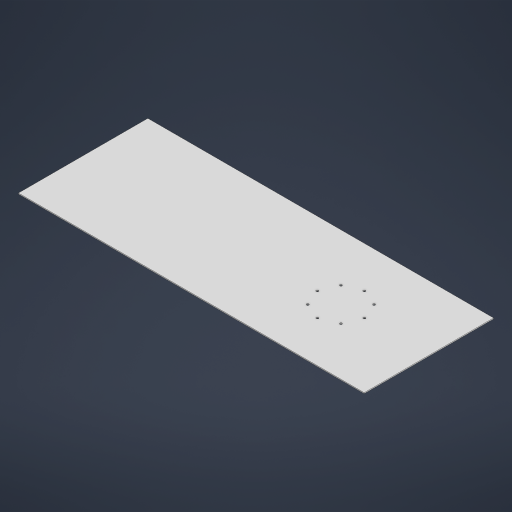
# Autodesk Inventor part: ChassisTop V3
Saved by Autodesk Inventor 2024 (Build 280153000, 153)
## iProperties
Created: 2023-11-20
Part Number: ChassisTop V3
Material: Generic
Document SubType Name: Modeling
Designer: avsar
Density: 1 g/cm^3
Appearance: Default
Author: avsar
Autodesk Inventor part; units mm, degrees
ref_plane "YZ Plane" through (0, 0, 0) normal (1, 0, 0) x (0, 1, 0)
ref_plane "XZ Plane" through (0, 0, 0) normal (0, 1, 0) x (-1, 0, 0)
ref_plane "XY Plane" through (0, 0, 0) normal (0, 0, 1) x (1, 0, 0)
sketch "Sketch1" plane through (0, 0, 0) normal (0, 1, 0) x (-1, 0, 0)
  line L0 (-305.435, 114.3) -> (305.435, 114.3)
  line L1 (305.435, 114.3) -> (305.435, -114.3)
  line L2 (305.435, -114.3) -> (-305.435, -114.3)
  line L3 (-305.435, -114.3) -> (-305.435, 114.3)
  line L4 (-305.435, 114.3) -> (305.435, -114.3) construction
  line L5 (305.435, 114.3) -> (-305.435, -114.3) construction
  point P0 (0, 0)
  dimension "d0" = 610.87
  dimension "d1" = 228.6
  constraints: 12 end point, 2 midpoint, 2 parallel, 1 horizontal, 1 perpendicular
  measures "d0" distance of L1.end L2.end
  measures "d1" distance of L0.end L1.end
extrude "Extrusion1" add sketch "Sketch1" along normal mid plane 1.5875
sketch "Sketch2" plane through (0, 0.7937, 0) normal (0, 1, 0) x (1, 0, 0)
  circle A0 centre (150, 0) radius 41.5 construction
  circle A1 centre (150, 41.5) radius 2
  circle A2 centre (120.6551, 29.3449) radius 2
  circle A3 centre (108.5, 0) radius 2
  circle A4 centre (120.6551, -29.3449) radius 2
  circle A5 centre (150, -41.5) radius 2
  circle A6 centre (179.3449, -29.3449) radius 2
  circle A7 centre (191.5, 0) radius 2
  circle A8 centre (179.3449, 29.3449) radius 2
  point P0 (0, 0)
  dimension "d4" = 83
  dimension "d5" = 150
  dimension "d6" = 4
  dimension "d9" = 360
  constraints: 8 centre point, 2 vertical alignment, 1 horizontal alignment, 19 other
  measures "d5" distance of point (150, 0) point (0, 0)
  measures "d6" diameter of A1
extrude "Extrusion2" cut sketch "Sketch2" against normal up to surface (1.5875 mm away)
body "Solid1"
